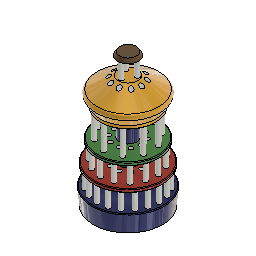
Cake v2 (Autodesk Fusion 360 design; units mm, degrees)
Autodesk Fusion 360 part; units mm, degrees
sketch "Sketch1" plane through (0, 0, 0) normal (0, 0, 1) x (1, 0, 0)
  circle A0 centre (0, 0) radius 25.4
  dimension "d1" = 50.8
  constraint coincident A0.centre origin
  measures "d1" diameter of A0
extrude "Extrude1" add sketch "Sketch1" along normal blind 12.7 draft 5 makes body 1
sketch "Sketch2" plane through (0, 0, 12.7) normal (0, 0, 1) x (-1, 0, 0)
  circle A0 centre (0, 0) radius 26.5111
  line L0 (0, 0) -> (0, 22.86) construction
  circle A1 centre (0, 22.86) radius 1.5875
  circle A2 centre (-7.0641, 21.7412) radius 1.5875
  line L1 (0, 0) -> (-7.0641, 21.7412) construction
  circle A3 centre (-13.4368, 18.4941) radius 1.5875
  line L2 (0, 0) -> (-13.4368, 18.4941) construction
  circle A4 centre (-18.4941, 13.4368) radius 1.5875
  line L3 (0, 0) -> (-18.4941, 13.4368) construction
  circle A5 centre (-21.7412, 7.0641) radius 1.5875
  line L4 (0, 0) -> (-21.7412, 7.0641) construction
  circle A6 centre (-22.86, 0) radius 1.5875
  line L5 (0, 0) -> (-22.86, 0) construction
  circle A7 centre (-21.7412, -7.0641) radius 1.5875
  line L6 (0, 0) -> (-21.7412, -7.0641) construction
  circle A8 centre (-18.4941, -13.4368) radius 1.5875
  line L7 (0, 0) -> (-18.4941, -13.4368) construction
  circle A9 centre (-13.4368, -18.4941) radius 1.5875
  line L8 (0, 0) -> (-13.4368, -18.4941) construction
  circle A10 centre (-7.0641, -21.7412) radius 1.5875
  line L9 (0, 0) -> (-7.0641, -21.7412) construction
  circle A11 centre (0, -22.86) radius 1.5875
  line L10 (0, 0) -> (0, -22.86) construction
  circle A12 centre (7.0641, -21.7412) radius 1.5875
  line L11 (0, 0) -> (7.0641, -21.7412) construction
  circle A13 centre (13.4368, -18.4941) radius 1.5875
  line L12 (0, 0) -> (13.4368, -18.4941) construction
  circle A14 centre (18.4941, -13.4368) radius 1.5875
  line L13 (0, 0) -> (18.4941, -13.4368) construction
  circle A15 centre (21.7412, -7.0641) radius 1.5875
  line L14 (0, 0) -> (21.7412, -7.0641) construction
  circle A16 centre (22.86, 0) radius 1.5875
  line L15 (0, 0) -> (22.86, 0) construction
  circle A17 centre (21.7412, 7.0641) radius 1.5875
  line L16 (0, 0) -> (21.7412, 7.0641) construction
  circle A18 centre (18.4941, 13.4368) radius 1.5875
  line L17 (0, 0) -> (18.4941, 13.4368) construction
  circle A19 centre (13.4368, 18.4941) radius 1.5875
  line L18 (0, 0) -> (13.4368, 18.4941) construction
  circle A20 centre (7.0641, 21.7412) radius 1.5875
  line L19 (0, 0) -> (7.0641, 21.7412) construction
  dimension "d4" = 22.86
  dimension "d5" = 3.175
  dimension "d7" = 360
  constraint coincident A0.centre L0.start
  constraint vertical L0
  constraint coincident L0.end A1.centre
  measures "d4" distance of A0.centre L0.end
  measures "d5" diameter of A1
extrude "Extrude2" add sketch "Sketch2" along normal blind 12.7 contours A1 | A2 | A3 | A4 | A5 | A6 | A7 | A8 | A9 | A10 | A11 | A12 | A13 | A14 | A15 | A16 | A17 | A18 | A19 | A20 bodies 1
sketch "Sketch3" plane through (0, 0, 25.4) normal (0, 0, 1) x (-1, 0, 0)
  circle A0 centre (-13.4368, 18.4941) radius 1.5875
  circle A1 centre (0, 0) radius 25.4
  dimension "d10" = 50.8
  constraint coincident A1.centre origin
  measures "d10" diameter of A1
extrude "Extrude3" add sketch "Sketch3" along normal blind 2.54 contours A0 | A1 bodies 1
sketch "Sketch4" plane through (0, 0, 27.94) normal (0, 0, 1) x (-1, 0, 0)
  circle A0 centre (0, 0) radius 25.4
  line L0 (0, 0) -> (0, 20.32) construction
  circle A1 centre (0, 20.32) radius 1.5875
  dimension "d13" = 20.32
  dimension "d14" = 3.175
  constraint coincident A0.centre L0.start
  constraint vertical L0
  constraint coincident L0.end A1.centre
  measures "d13" distance of A0.centre L0.end
  measures "d14" diameter of A1
extrude "Extrude4" add sketch "Sketch4" along normal blind 12.7 contours A1 bodies 1
pattern_circular "C-Pattern1" count 15 over 360 about axis through (0, 0, 25.4) along (0, 0, 1) of "Extrude4"
sketch "Sketch5" plane through (0, 0, 40.64) normal (0, 0, 1) x (-1, 0, 0)
  circle A0 centre (-8.2649, 18.5632) radius 1.5875
  circle A1 centre (0, 0) radius 22.86
  dimension "d19" = 45.72
  constraint coincident A1.centre origin
  measures "d19" diameter of A1
extrude "Extrude5" add sketch "Sketch5" along normal blind 2.54 contours A0 | A1 bodies 1
sketch "Sketch6" plane through (0, 0, 43.18) normal (0, 0, 1) x (-1, 0, 0)
  circle A0 centre (0, 0) radius 22.86
  line L0 (0, 0) -> (0, 17.78) construction
  circle A1 centre (0, 17.78) radius 1.5875
  dimension "d22" = 3.175
  dimension "d23" = 17.78
  constraint coincident A0.centre L0.start
  constraint vertical L0
  constraint coincident L0.end A1.centre
  measures "d22" diameter of A1
  measures "d23" distance of A0.centre L0.end
extrude "Extrude6" add sketch "Sketch6" along normal blind 19.05 contours A1 bodies 1
pattern_circular "C-Pattern2" count 10 over 360 about axis through (0, 0, 43.18) along (0, 0, 1) of "Extrude6"
sketch "Sketch7" plane through (0, 0, 62.23) normal (0, 0, 1) x (-1, 0, 0)
  circle A0 centre (0, 17.78) radius 1.5875
  circle A1 centre (0, 0) radius 20.32
  dimension "d28" = 40.64
  constraint coincident A1.centre origin
  measures "d28" diameter of A1
extrude "Extrude7" add sketch "Sketch7" along normal blind 2.54 separate body contours A0 | A1 makes body 2
sketch "Sketch8" plane through (0, 0, 64.77) normal (0, 0, 1) x (-1, 0, 0)
  circle A0 centre (0, 0) radius 20.32
  circle A1 centre (0, 0) radius 20.32
  constraint coincident A0.centre A1.centre
extrude "Extrude8" add sketch "Sketch8" along normal blind 7.62 draft 30 bodies 2
sketch "Sketch9" plane through (0, 0, 72.39) normal (0, 0, 1) x (-1, 0, 0)
  circle A0 centre (0, 0) radius 24.7194
  circle A1 centre (0, 0) radius 24.7194
  constraint coincident A0.centre A1.centre
extrude "Extrude9" add sketch "Sketch9" along normal blind 10.16 draft -60 bodies 2
sketch "Sketch10" plane through (0, 0, 82.55) normal (0, 0, 1) x (-1, 0, 0)
  circle A0 centre (0, 0) radius 7.1218
  line L0 (0, 0) -> (0, 5.08) construction
  circle A1 centre (0, 5.08) radius 1.5875
  dimension "d35" = 3.175
  dimension "d36" = 5.08
  constraint coincident A0.centre L0.start
  constraint vertical L0
  constraint coincident L0.end A1.centre
  measures "d35" diameter of A1
  measures "d36" distance of A0.centre L0.end
extrude "Extrude10" add sketch "Sketch10" along normal blind 12.7 contours A1 bodies 2
pattern_circular "C-Pattern3" count 3 over 360 about axis through (0, 0, 82.55) along (0, 0, -1) of "Extrude10"
sketch "Sketch11" plane through (0, 0, 95.25) normal (0, 0, 1) x (-1, 0, 0)
  circle A0 centre (0, 5.08) radius 1.5875
  circle A1 centre (0, 0) radius 7.62
  dimension "d41" = 15.24
  constraint coincident A1.centre origin
  measures "d41" diameter of A1
extrude "Extrude11" add sketch "Sketch11" along normal blind 2.54 draft -30 contours A0 | A1 bodies 2
fillet "Fillet1" radius 0.508 6 edges at (21.313, 8.2665, 43.18) (21.313, 8.2665, 40.64) (23.6811, 9.185, 27.94) (23.6811, 9.185, 25.4) (-24.717, 9.5868, 12.7) (18.9449, 7.348, 62.23) on bodies 1 2
fillet "Fillet2" radius 2.54 1 edges at (23.0466, -8.9389, 72.39) on bodies 2
sketch "Sketch12" plane through (0, 0, 12.7) normal (0, 0, 1) x (-1, 0, 0)
  circle A0 centre (0, -22.86) radius 1.5875
  circle A1 centre (-21.7412, -7.0641) radius 1.5875
  circle A2 centre (-13.4368, 18.4941) radius 1.5875
  circle A3 centre (21.7412, 7.0641) radius 1.5875
  circle A4 centre (0, 22.86) radius 1.5875
  circle A5 centre (7.0641, 21.7412) radius 1.5875
  circle A6 centre (22.86, 0) radius 1.5875
  circle A7 centre (-18.4941, 13.4368) radius 1.5875
  circle A8 centre (-18.4941, -13.4368) radius 1.5875
  circle A9 centre (7.0641, -21.7412) radius 1.5875
  circle A10 centre (-7.0641, -21.7412) radius 1.5875
  circle A11 centre (-22.86, 0) radius 1.5875
  circle A12 centre (18.4941, -13.4368) radius 1.5875
  circle A13 centre (18.4941, 13.4368) radius 1.5875
  circle A14 centre (-7.0641, 21.7412) radius 1.5875
  circle A15 centre (13.4368, 18.4941) radius 1.5875
  circle A16 centre (21.7412, -7.0641) radius 1.5875
  circle A17 centre (-21.7412, 7.0641) radius 1.5875
  circle A18 centre (-13.4368, -18.4941) radius 1.5875
  circle A19 centre (13.4368, -18.4941) radius 1.5875
  circle A20 centre (0, 0) radius 25.9567
  circle A21 centre (0, 0) radius 6.35
  dimension "d48" = 12.7
  constraint coincident A20.centre A21.centre
  measures "d48" diameter of A21
extrude "Extrude12" add sketch "Sketch12" along normal up to surface (49.53 mm away) contours A21 bodies 1 2
sketch "Sketch13" plane through (0, 0, 12.7) normal (0, 0, 1) x (-1, 0, 0)
  circle A0 centre (0, 0) radius 6.35
  circle A1 centre (0, -22.86) radius 1.5875
  circle A2 centre (-21.7412, -7.0641) radius 1.5875
  circle A3 centre (-13.4368, 18.4941) radius 1.5875
  circle A4 centre (21.7412, 7.0641) radius 1.5875
  circle A5 centre (0, 22.86) radius 1.5875
  circle A6 centre (7.0641, 21.7412) radius 1.5875
  circle A7 centre (22.86, 0) radius 1.5875
  circle A8 centre (-18.4941, 13.4368) radius 1.5875
  circle A9 centre (-18.4941, -13.4368) radius 1.5875
  circle A10 centre (7.0641, -21.7412) radius 1.5875
  circle A11 centre (-7.0641, -21.7412) radius 1.5875
  circle A12 centre (-22.86, 0) radius 1.5875
  circle A13 centre (18.4941, -13.4368) radius 1.5875
  circle A14 centre (18.4941, 13.4368) radius 1.5875
  circle A15 centre (-7.0641, 21.7412) radius 1.5875
  circle A16 centre (13.4368, 18.4941) radius 1.5875
  circle A17 centre (21.7412, -7.0641) radius 1.5875
  circle A18 centre (-21.7412, 7.0641) radius 1.5875
  circle A19 centre (-13.4368, -18.4941) radius 1.5875
  circle A20 centre (13.4368, -18.4941) radius 1.5875
  circle A21 centre (0, 0) radius 25.9567
  line L0 (0, 0) -> (-10.16, 0) construction
  circle A22 centre (-10.16, 0) radius 1.5875
  circle A23 centre (-8.2196, -5.9719) radius 1.5875
  line L1 (0, 0) -> (-8.2196, -5.9719) construction
  circle A24 centre (-3.1396, -9.6627) radius 1.5875
  line L2 (0, 0) -> (-3.1396, -9.6627) construction
  circle A25 centre (3.1396, -9.6627) radius 1.5875
  line L3 (0, 0) -> (3.1396, -9.6627) construction
  circle A26 centre (8.2196, -5.9719) radius 1.5875
  line L4 (0, 0) -> (8.2196, -5.9719) construction
  circle A27 centre (10.16, 0) radius 1.5875
  line L5 (0, 0) -> (10.16, 0) construction
  circle A28 centre (8.2196, 5.9719) radius 1.5875
  line L6 (0, 0) -> (8.2196, 5.9719) construction
  circle A29 centre (3.1396, 9.6627) radius 1.5875
  line L7 (0, 0) -> (3.1396, 9.6627) construction
  circle A30 centre (-3.1396, 9.6627) radius 1.5875
  line L8 (0, 0) -> (-3.1396, 9.6627) construction
  circle A31 centre (-8.2196, 5.9719) radius 1.5875
  line L9 (0, 0) -> (-8.2196, 5.9719) construction
  dimension "d51" = 10.16
  dimension "d52" = 3.175
  dimension "d54" = 360
  constraint coincident A0.centre A21.centre
  constraint horizontal L0
  constraint coincident L0.end A22.centre
  measures "d51" distance of A0.centre L0.end
  measures "d52" diameter of A22
extrude "Extrude13" cut sketch "Sketch13" along normal through all contours A22 | A23 | A24 | A25 | A26 | A27 | A28 | A29 | A30 | A31 bodies 1
